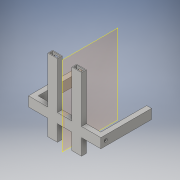
# Autodesk Inventor part: Shooter
Saved by Autodesk Inventor 2016 SP1 (Build 200210100, 210)
## iProperties
Created: 2016-02-06
Part Number: Shooter
Material: Generic
Document SubType Name: Modeling
Designer: steele
Density: 1 g/cm^3
Appearance: Default
Author: steele
Autodesk Inventor part; units mm, degrees
ref_plane "XZ Plane" through (0, 0, 0) normal (0, 1, 0) x (-1, 0, 0)
sketch "Sketch1" plane through (0, 0, 0) normal (0, 1, 0) x (-1, 0, 0)
  line L0 (0, 0) -> (133.35, 0)
  line L1 (133.35, 0) -> (133.35, -190.5)
  line L2 (0, 0) -> (0, -190.5) construction
  line L3 (0, 0) -> (-133.35, 0)
  line L4 (-133.35, 0) -> (-133.35, -190.5)
  dimension "d0" = 133.35
  dimension "d1" = 190.5
  dimension "d2" = 190.5
  constraints: 10 end point, 2 symmetric about line, 1 horizontal, 1 perpendicular, 1 vertical
  measures "d0" distance of L0.start L0.end
  measures "d1" distance of L0.end L1.end
  measures "d2" distance of L0.start L2.end
ref_plane "Work Plane1" through (0, 0, -190.5) normal (0, 0, 1) x (1, 0, 0)
sketch "Sketch3" plane through (0, 0, -190.5) normal (0, 0, 1) x (1, 0, 0)
  line L0 (142.875, -19.05) -> (123.825, -19.05)
  line L1 (123.825, -19.05) -> (123.825, 19.05)
  line L2 (123.825, 19.05) -> (142.875, 19.05)
  line L3 (142.875, 19.05) -> (142.875, -19.05)
  line L4 (142.875, -19.05) -> (123.825, 19.05) construction
  line L5 (123.825, -19.05) -> (142.875, 19.05) construction
  line L6 (139.7, -15.875) -> (127, -15.875)
  line L7 (127, -15.875) -> (127, 15.875)
  line L8 (127, 15.875) -> (139.7, 15.875)
  line L9 (139.7, 15.875) -> (139.7, -15.875)
  line L10 (139.7, -15.875) -> (127, 15.875) construction
  line L11 (127, -15.875) -> (139.7, 15.875) construction
  point P0 (0, 0)
  point P1 (133.35, 0)
  dimension "d4" = 38.1
  dimension "d5" = 19.05
  dimension "d6" = 133.35
  dimension "d7" = 3.175
  dimension "d8" = 3.175
  constraints: 24 end point, 4 midpoint, 4 parallel, 2 horizontal, 2 perpendicular
  measures "d4" distance of L2.end L0.start
  measures "d5" distance of L0.start L0.end
  measures "d6" distance of point (133.35, 0) point (0, 0)
  measures "d7" distance between parallel lines of L2 L8
  measures "d8" distance between parallel lines of L3 L9
sweep "Sweep1" add profiles "Sketch3" path "Sketch1"
sketch "Sketch4" plane through (123.825, 19.05, -190.5) normal (0, 1, 0) x (1, 0, 0)
  line L0 (-190.5, -200.025) -> (-152.4, -200.025)
  line L1 (-152.4, -200.025) -> (-152.4, -180.975)
  line L2 (-152.4, -180.975) -> (-190.5, -180.975)
  line L3 (-190.5, -180.975) -> (-190.5, -200.025)
  line L4 (-190.5, -200.025) -> (-152.4, -180.975) construction
  line L5 (-152.4, -200.025) -> (-190.5, -180.975) construction
  line L6 (-266.7, -200.025) -> (-266.7, 0) projected
  line L7 (-187.325, -196.85) -> (-155.575, -196.85)
  line L8 (-155.575, -196.85) -> (-155.575, -184.15)
  line L9 (-155.575, -184.15) -> (-187.325, -184.15)
  line L10 (-187.325, -184.15) -> (-187.325, -196.85)
  line L11 (-187.325, -196.85) -> (-155.575, -184.15) construction
  line L12 (-155.575, -196.85) -> (-187.325, -184.15) construction
  line L13 (3.175, -184.15) -> (-250.825, -184.15) projected
  point P0 (-123.825, -190.5)
  point P1 (-171.45, -190.5)
  dimension "d11" = 95.25
  dimension "d12" = 19.05
  dimension "d13" = 38.1
  dimension "d14" = 3.175
  dimension "d15" = 3.175
  constraints: 24 end point, 5 parallel, 4 midpoint, 2 perpendicular, 1 horizontal
  measures "d11" distance from line of point (-171.45, -190.5) L6
  measures "d12" distance of L2.end L0.start
  measures "d13" distance of L0.start L0.end
  measures "d14" distance between parallel lines of L10 L3
  measures "d15" distance between parallel lines of L0 L7
extrude "Extrusion1" add sketch "Sketch4" along normal blind 184.15 contours L3 L13 L10 L7 L8 L1 L0 | L3 L2 L1 L13 L9
sketch "Sketch5" plane through (123.825, -19.05, -190.5) normal (0, -1, 0) x (1, 0, 0)
  line L0 (-190.5, 180.975) -> (-152.4, 180.975)
  line L1 (-152.4, 180.975) -> (-152.4, 200.025)
  line L2 (-152.4, 200.025) -> (-190.5, 200.025)
  line L3 (-190.5, 200.025) -> (-190.5, 180.975)
  line L4 (-190.5, 180.975) -> (-152.4, 200.025) construction
  line L5 (-152.4, 180.975) -> (-190.5, 200.025) construction
  line L6 (-266.7, 200.025) -> (-266.7, 0) projected
  line L7 (-187.325, 184.15) -> (-155.575, 184.15)
  line L8 (-155.575, 184.15) -> (-155.575, 196.85)
  line L9 (-155.575, 196.85) -> (-187.325, 196.85)
  line L10 (-187.325, 196.85) -> (-187.325, 184.15)
  line L11 (-187.325, 184.15) -> (-155.575, 196.85) construction
  line L12 (-155.575, 184.15) -> (-187.325, 196.85) construction
  point P0 (-123.825, 190.5)
  point P1 (-171.45, 190.5)
  dimension "d18" = 95.25
  dimension "d19" = 19.05
  dimension "d20" = 38.1
  dimension "d21" = 3.175
  dimension "d22" = 3.175
  constraints: 24 end point, 4 midpoint, 4 parallel, 2 horizontal, 2 perpendicular
  measures "d18" distance from line of point (-171.45, 190.5) L6
  measures "d19" distance of L2.end L0.start
  measures "d20" distance of L1.end L2.end
  measures "d21" distance between parallel lines of L9 L2
  measures "d22" distance between parallel lines of L3 L10
extrude "Extrusion2" add sketch "Sketch5" along normal blind 63.5
mirror "Mirror1" about plane through (0, 0, 0) normal (1, 0, 0) of "Extrusion1", "Extrusion2"
sketch "Sketch6" plane through (142.875, -19.05, -190.5) normal (1, 0, 0) x (0, 0, -1)
  line L0 (-200.025, 0) -> (-200.025, 38.1) projected
  point P0 (-190.5, 19.05)
  point P1 (-180.975, 19.05)
  dimension "d25" = 19.05
  measures "d25" distance from line of L0 point (-180.975, 19.05)
hole "Hole1" at (142.875, 0, -9.525) direction (-1, 0, 0) diameter 12.7 depth 3.175 tip angle 118
sketch "Sketch7" plane through (-66.675, 19.05, -9.525) normal (0, 0, -1) x (-1, 0, 0)
  line L0 (-38.1, 184.15) -> (0, 184.15) construction
  line L1 (-19.05, 184.15) -> (-19.05, -101.6) construction
  line L2 (-34.925, -101.6) -> (-3.175, -101.6) construction
  line L3 (-95.25, 184.15) -> (-133.35, 184.15) construction
  line L4 (-114.3, 184.15) -> (-114.3, -101.6) construction
  line L5 (-133.35, -101.6) -> (-95.25, -101.6) construction
  point P0 (-66.675, -19.05)
  point P1 (-19.05, 165.1)
  point P2 (-19.05, -82.55)
  point P3 (-114.3, -82.55)
  point P4 (-114.3, 165.1)
  dimension "d33" = 19.05
  dimension "d34" = 19.05
  dimension "d35" = 19.05
  dimension "d36" = 19.05
  constraints: 4 end point, 4 midpoint, 4 point on line
  measures "d33" distance from line of L0 point (-19.05, 165.1)
  measures "d34" distance from line of L3 point (-114.3, 165.1)
  measures "d35" distance of L1.end point (-19.05, -82.55)
  measures "d36" distance from line of point (-114.3, -82.55) L5
hole "Hole2" at (-47.625, 184.15, -9.525) at (-47.625, -63.5, -9.525) at (47.625, -63.5, -9.525) at (47.625, 184.15, -9.525) direction (0, 0, 1) diameter 25.4 depth 3.175 tip angle 118
mirror "Mirror2" about plane through (0, 0, 0) normal (1, 0, 0) of "Hole1"
equation "\"d0\" = 0.5 * width"
equation "\"d1\" = length"
equation "\"d2\" = length"
equation "\"d4\" = tubingLength"
equation "\"d5\" = tubingWidth"
equation "\"d6\" = 0.5 * width"
equation "\"d7\" = tubeingWallWidth"
equation "\"d8\" = tubeingWallWidth"
equation "\"d12\" = tubingWidth"
equation "\"d13\" = tubingLength"
equation "\"d14\" = tubeingWallWidth"
equation "\"d15\" = tubeingWallWidth"
equation "\"d19\" = tubingWidth"
equation "\"d20\" = tubingLength"
equation "\"d21\" = tubeingWallWidth"
equation "\"d22\" = tubeingWallWidth"
equation "\"width\" = 266.7"
equation "\"length\" = 190.5"
equation "\"tubingWidth\" = 19.05"
equation "\"tubingLength\" = 38.1"
equation "\"tubeingWallWidth\" = 3.175"
equation "\"d3\" = -length"
body "Solid1"
